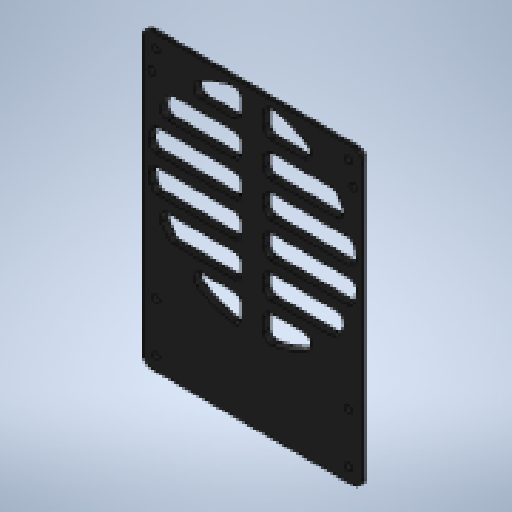
# Autodesk Inventor part: Face Plate
Saved by Autodesk Inventor 2023.2 (Build 272271000, 271)
## iProperties
Created: 2023-08-15
Part Number: Face Plate
Material: UHMW, Black
Document SubType Name: Modeling
Designer: Nathan Cai
Density: 0.94 g/cm^3
Appearance: Smooth - Black
Author: Nathan Cai
Autodesk Inventor part; units mm, degrees
ref_plane "YZ Plane" through (0, 0, 0) normal (1, 0, 0) x (0, 1, 0)
ref_plane "XZ Plane" through (0, 0, 0) normal (0, 1, 0) x (-1, 0, 0)
ref_plane "XY Plane" through (0, 0, 0) normal (0, 0, 1) x (1, 0, 0)
sketch "Sketch1" plane through (0, 0, 0) normal (0, 0, 1) x (1, 0, 0)
  line L0 (-60, -80) -> (60, -80)
  line L1 (60, -80) -> (60, 80)
  line L2 (60, 80) -> (-60, 80)
  line L3 (-60, 80) -> (-60, -80)
  line L4 (-60, -80) -> (60, 80) construction
  line L5 (60, -80) -> (-60, 80) construction
  line L6 (0, 80) -> (0, -80) construction
  line L7 (-52.5, 72.5) -> (52.5, 72.5) construction
  line L8 (52.5, 72.5) -> (52.5, -32.5) construction
  line L9 (52.5, -32.5) -> (-52.5, -32.5) construction
  line L10 (-52.5, -32.5) -> (-52.5, 72.5) construction
  line L11 (-52.5, 72.5) -> (52.5, -32.5) construction
  line L12 (52.5, 72.5) -> (-52.5, -32.5) construction
  circle A0 centre (-52.5, 72.5) radius 2
  circle A1 centre (52.5, 72.5) radius 2
  circle A2 centre (-52.5, -32.5) radius 2
  circle A3 centre (52.5, -32.5) radius 2
  circle A4 centre (-52.5, -72.5) radius 2
  circle A5 centre (52.5, -72.5) radius 2
  circle A6 centre (0, 20) radius 57
  circle A7 centre (52.5, -45.5) radius 2
  circle A8 centre (-52.5, -45.5) radius 2
  circle A9 centre (55, 61) radius 2
  circle A10 centre (-55, 61) radius 2
  point P0 (0, 0)
  point P1 (0, 20)
  dimension "d0" = 120
  dimension "d1" = 160
  dimension "d2" = 105
  dimension "d4" = 7.5
  dimension "d5" = 4
  dimension "d8" = 105
  dimension "d11" = 105
  dimension "d16" = 40
  dimension "d21" = 114
  dimension "d82" = 13
  dimension "d122" = 47.5
  dimension "d130" = 19
  dimension "d131" = 5
  dimension "d132" = 4
  constraints: 26 end point, 11 centre point, 6 midpoint, 4 parallel, 3 horizontal, 3 vertical, 2 coincident, 2 perpendicular, 1 point on line, 1 symmetric about line, 15 other
  measures "d0" distance of L2.end L1.end
  measures "d1" distance of L1.end L0.end
  measures "d2" distance of L8.end L9.end
  measures "d4" distance between parallel lines of L2 L7
  measures "d5" diameter of A0
  measures "d8" distance of A0.centre A1.centre
  measures "d11" distance of A0.centre A2.centre
  measures "d16" distance of A2.centre A4.centre
  measures "d21" diameter of A6
  measures "d82" distance of A3.centre A7.centre
  measures "d122" distance between parallel lines of L0 L9
  measures "d130" distance from line of L2 A9.centre
  measures "d131" distance from line of L1 A9.centre
  measures "d132" diameter of A9
extrude "Extrusion1" add sketch "Sketch1" along normal blind 4 contours L3 L2 L1 L0 | A2 | A3
sketch "Sketch2" plane through (0, 0, 4) normal (0, 0, 1) x (1, 0, 0)
  line L0 (60, -80) -> (60, 80) projected
  line L1 (60, 80) -> (-60, 80) projected
  line L2 (-60, 80) -> (-60, -80) projected
  line L3 (-60, -80) -> (60, -80) projected
  circle A0 centre (-52.5, -72.5) radius 2 projected
  circle A1 centre (52.5, -72.5) radius 2 projected
  circle A2 centre (0, 20) radius 57 projected
  circle A3 centre (52.5, 72.5) radius 2 projected
  circle A4 centre (-52.5, 72.5) radius 2 projected
  line L4 (0, 73.4838) -> (0, -23.4838) construction
  line L5 (-6, 77) -> (6, 77) construction
  line L6 (6, 77) -> (6, -37)
  line L7 (6, -37) -> (-6, -37) construction
  line L8 (-6, -37) -> (-6, 77)
  line L9 (-6, 77) -> (6, -37) construction
  line L10 (6, 77) -> (-6, -37) construction
  circle A5 centre (0, 20) radius 57 projected
  line L11 (-44.9889, 61) -> (44.9889, 61)
  line L12 (44.9889, 61) -> (44.9889, 55)
  line L13 (44.9889, 55) -> (-44.9889, 55)
  line L14 (-44.9889, 55) -> (-44.9889, 61)
  line L15 (-44.9889, 61) -> (44.9889, 55) construction
  line L16 (44.9889, 61) -> (-44.9889, 55) construction
  line L17 (-57, 17) -> (57, 17)
  line L18 (57, 17) -> (57, 23)
  line L19 (57, 23) -> (-57, 23)
  line L20 (-57, 23) -> (-57, 17)
  line L21 (-57, 17) -> (57, 23) construction
  line L22 (57, 17) -> (-57, 23) construction
  line L23 (-54.7083, 42) -> (54.7083, 42)
  line L24 (54.7083, 42) -> (54.7083, 36)
  line L25 (54.7083, 36) -> (-54.7083, 36)
  line L26 (-54.7083, 36) -> (-54.7083, 42)
  line L27 (-54.7083, 42) -> (54.7083, 36) construction
  line L28 (54.7083, 42) -> (-54.7083, 36) construction
  line L29 (-57, 20) -> (57, 20) construction
  line L30 (-44.9889, -21) -> (44.9889, -21)
  line L31 (44.9889, -21) -> (44.9889, -15)
  line L32 (44.9889, -15) -> (-44.9889, -15)
  line L33 (-44.9889, -15) -> (-44.9889, -21)
  line L34 (-44.9889, -21) -> (44.9889, -15) construction
  line L35 (44.9889, -21) -> (-44.9889, -15) construction
  line L36 (-54.7083, -2) -> (54.7083, -2)
  line L37 (54.7083, -2) -> (54.7083, 4)
  line L38 (54.7083, 4) -> (-54.7083, 4)
  line L39 (-54.7083, 4) -> (-54.7083, -2)
  line L40 (-54.7083, -2) -> (54.7083, 4) construction
  line L41 (54.7083, -2) -> (-54.7083, 4) construction
  point P0 (0, 58)
  point P1 (0, 39)
  point P2 (0, -18)
  point P3 (0, 1)
  point P4 (6, 61)
  point P5 (6, 76.6833)
  point P6 (-6, 76.6833)
  point P7 (-6, 61)
  point P8 (-39.598, 61)
  point P9 (-44.9889, 55)
  point P10 (-6, 55)
  point P11 (-6, 42)
  point P12 (-52.5833, 42)
  point P13 (-6, 36)
  point P14 (-6, 23)
  point P15 (-56.921, 23)
  point P16 (-56.921, 17)
  point P17 (-6, 17)
  point P18 (-6, 4)
  point P19 (-54.7083, 4)
  point P20 (-52.5833, -2)
  point P21 (-6, -2)
  point P22 (-6, -15)
  point P23 (-44.9889, -15)
  point P24 (-39.598, -21)
  point P25 (-6, -21)
  point P26 (-6, -36.6833)
  point P27 (6, -36.6833)
  point P28 (6, -21)
  point P29 (39.598, -21)
  point P30 (44.9889, -15)
  point P31 (6, -15)
  point P32 (6, -2)
  point P33 (52.5833, -2)
  point P34 (54.7083, 4)
  point P35 (6, 4)
  point P36 (6, 17)
  point P37 (56.921, 17)
  point P38 (56.921, 23)
  point P39 (6, 23)
  point P40 (6, 36)
  point P41 (54.7083, 36)
  point P42 (52.5833, 42)
  point P43 (6, 42)
  point P44 (6, 55)
  point P45 (44.9889, 55)
  point P46 (39.598, 61)
  dimension "d106" = 12
  dimension "d108" = 6
  dimension "d110" = 35
  dimension "d111" = 6
  dimension "d112" = 6
  dimension "d113" = 13
  constraints: 76 end point, 10 midpoint, 10 symmetric about line, 8 parallel, 6 horizontal, 4 perpendicular, 4 point on line, 2 vertical, 4 other
  measures "d106" distance of L6.end L7.end
  measures "d108" distance of L11.end L12.end
  measures "d110" distance from line of point (0, 20) L13
  measures "d111" distance between parallel lines of L19 L17
  measures "d112" distance between parallel lines of L25 L23
  measures "d113" distance between parallel lines of L19 L25
extrude "Extrusion2" add sketch "Sketch2" against normal up to surface (4 mm away) contours A2 L17 L6 L19 | L25 L6 L23 A2 | L19 L8 L25 L6 | L6 L17 L8 L19 | A2 L36 L6 L38 | L6 L38 L8 L17 | L25 L8 L23 L6 | L8 L17 A2 L19 | L6 L36 L8 L38 | L13 L6 L11 A2 | L23 L8 L13 L6 | L25 A2 L23 L8 | A2 L30 L6 L32 | L6 L32 L8 L36 | L8 L36 A2 L38 | L13 L8 L11 L6 | L6 L30 L8 L32 | L6 L11 L8 A2 | L13 A2 L11 L8 | A2 L8 L30 L6 | L8 L30 A2 L32
fillet "Fillet4" radius 4 44 edges at (-44.9889, -15, 2) (44.9889, -15, 2) (-39.598, -21, 2) (39.598, -21, 2) (6, 76.6833, 2) (6, -36.6833, 2) (6, -21, 2) (6, -15, 2) (-6, -15, 2) (-6, 76.6833, 2) (-6, -36.6833, 2) (-6, -21, 2) (-52.5833, -2, 2) (52.5833, -2, 2) (-6, -2, 2) (6, -2, 2) (-54.7083, 4, 2) (54.7083, 4, 2) (6, 4, 2) (-6, 4, 2) (-56.921, 17, 2) (56.921, 17, 2) (56.921, 23, 2) (-56.921, 23, 2) (-6, 23, 2) (-6, 17, 2) (6, 17, 2) (6, 23, 2) (54.7083, 36, 2) (-54.7083, 36, 2) (6, 36, 2) (-6, 36, 2) (52.5833, 42, 2) (-52.5833, 42, 2) (-6, 42, 2) (-6, 55, 2) (44.9889, 55, 2) (-44.9889, 55, 2) (39.598, 61, 2) (-39.598, 61, 2) (-6, 61, 2) (6, 61, 2) (6, 55, 2) (6, 42, 2)
fillet "Fillet1" radius 5 4 edges at (60, 80, 2) (-60, -80, 2) (-60, 80, 2) (60, -80, 2)
chamfer "Chamfer2" distance 2 angle 45 8 edges at (60, 0, 0) (58.5355, 78.5355, 0) (0, 80, 0) (-58.5355, 78.5355, 0) (-60, 0, 0) (-58.5355, -78.5355, 0) (0, -80, 0) (58.5355, -78.5355, 0)
equation "\"d8\" = d3"
equation "\"d11\" = d2"
equation "\"d111\" = d108"
equation "\"d112\" = d108"
equation "\"d3\" = 105"
body "Solid1"
